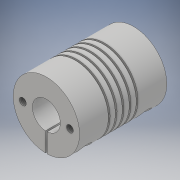
# Autodesk Inventor part: Муфта4х5
Saved by Autodesk Inventor 2017 (Build 210142000, 142)
## iProperties
Part Number: Муфта4х5
Material: Типовые
Document SubType Name: Modeling
Designer: Daemon
Density: 1 g/cm^3
Appearance: По умолчанию
Author: Daemon
Autodesk Inventor part; units mm, degrees
sketch "Эскиз1" plane through (0, 0, 0) normal (0, 0, 1) x (1, 0, 0)
  circle A0 centre (0, 0) radius 9.5
  dimension "d0" = 19
  constraints: 1 centre point, 1 coincident
  measures "d0" diameter of A0
extrude "Выдавливание1" add sketch "Эскиз1" along normal blind 25
sketch "Эскиз2" plane through (0, 0, 25) normal (0, 0, 1) x (1, 0, 0)
  circle A0 centre (0, 0) radius 3
  dimension "d3" = 6
  constraints: 1 centre point, 1 coincident
  measures "d3" diameter of A0
extrude "Выдавливание2" cut sketch "Эскиз2" against normal blind 12.5
sketch "Эскиз3" plane through (0, 0, 0) normal (0, 0, -1) x (-1, 0, 0)
  circle A0 centre (0, 0) radius 4
  dimension "d6" = 8
  constraints: 1 centre point, 1 coincident
  measures "d6" diameter of A0
extrude "Выдавливание3" cut sketch "Эскиз3" against normal blind 12.5
ref_plane "РабПлоскость1" through (-9.5, 0, 0) normal (1, 0, 0) x (0, 1, 0)
ref_plane "РабПлоскость2" through (0, 0, 12.5) normal (0, 0, -1) x (-1, 0, 0)
sketch "Эскиз5" plane through (0, 0, 12.5) normal (0, 0, -1) x (-1, 0, 0)
  circle A0 centre (0, 0) radius 9.5
  circle A1 centre (0, 0) radius 6.75
  dimension "d20" = 19
  dimension "d21" = 13.5
  constraints: 2 centre point, 2 coincident
  measures "d20" diameter of A0
  measures "d21" diameter of A1
extrude "Выдавливание5" cut sketch "Эскиз5" along normal mid plane 0.5
pattern_linear "Прямоуг.массив2" count 3 spacing 2 along (0, 0, 1) of "Выдавливание5"
pattern_linear "Прямоуг.массив3" count 3 spacing 2 along (0, 0, -1) of "Выдавливание5"
sketch "Эскиз6" plane through (0, 0, 0) normal (0, 0, -1) x (-1, 0, 0)
  circle A0 centre (0, 0) radius 9.5 projected
  circle A1 centre (0, 0) radius 6.75 projected
  line L0 (-9.5, 0.25) -> (-9.5, 0)
  line L1 (2, 0) -> (2, 0.25)
  line L2 (2, 0.25) -> (-9.5, 0.25)
  line L3 (2, 0) -> (-9.5, 0)
  dimension "d49" = 11.5
  dimension "d50" = 0.25
  constraints: 8 end point, 1 horizontal, 1 horizontal alignment, 1 perpendicular, 1 other
  measures "d49" distance of L1.start L0.end
  measures "d50" distance of L1.start L1.end
extrude "Выдавливание6" cut sketch "Эскиз6" against normal up to next contours L0 L2 A0 | A0 L2 A1 L3 | A1 L2 L1 L3 picked at (-7.6653, 0.1389) picked at (-0.9151, 0.1667)
sketch "Эскиз7" plane through (0, 0, 0) normal (0, 0, -1) x (-1, 0, 0)
  arc A0 (-6.75, 0) -> (-6.7454, 0.25) centre (0, 0) ccw projected
  circle A1 centre (0, 6.75) radius 1
  point P0 (6.7454, 0.25)
  dimension "d33" = 2
  constraints: 1 centre point, 1 point on circle
  measures "d33" diameter of A1
extrude "Выдавливание7" cut sketch "Эскиз7" against normal blind 4
pattern_circular "Круговой массив2" count 2 over 360 about axis through (0, 0, 0) along (0, 0, 1) of "Выдавливание7"
mirror "Зеркальное отражение2" about plane through (0, 0, 12.5) normal (0, 0, -1) of "Выдавливание7", "Круговой массив2"
thread "Резьба1" size "M2x0.4" class "6H" standard "ANSI Metric M Profile" full length
thread "Резьба2" size "M2x0.4" class "6H" standard "ANSI Metric M Profile" full length
thread "Резьба3" size "M2x0.4" class "6H" standard "ANSI Metric M Profile" full length
thread "Резьба4" size "M2x0.4" class "6H" standard "ANSI Metric M Profile" full length
mirror "Зеркальное отражение3" about plane through (-2, 0, 0) normal (0, 1, 0) of "Выдавливание6"
ref_plane "РабПлоскость3" through (0, -9.5, 0) normal (0, 1, 0) x (-1, 0, 0)
sketch "Эскиз8" plane through (0, -9.5, 0) normal (0, 1, 0) x (-1, 0, 0)
  line L0 (-9.5, -0.0521) -> (-9.5, 3.9479)
  line L1 (-9.5, 3.9479) -> (-7, 3.9479)
  circle A0 centre (-7, 3.9479) radius 1
  point P0 (0, 0)
  dimension "d51" = 2
  dimension "d52" = 2.5
  dimension "d53" = 4
  constraints: 4 end point, 1 centre point, 1 coincident, 1 horizontal, 1 vertical
  measures "d51" diameter of A0
  measures "d52" distance of L0.end L1.end
  measures "d53" distance of L0.start L0.end
extrude "Выдавливание8" cut sketch "Эскиз8" along normal up to next
sketch "Эскиз9" plane through (0, -9.5, 0) normal (0, 1, 0) x (-1, 0, 0)
  circle A0 centre (-7, 3.9479) radius 1 projected
  circle A1 centre (-7, 3.9479) radius 2
  point P0 (0, 0)
  dimension "d56" = 4
  constraints: 1 centre point, 1 coincident
  measures "d56" diameter of A1
extrude "Выдавливание9" cut sketch "Эскиз9" along normal blind 5
ref_plane "РабПлоскость5" through (0, 9.5, 0) normal (0, 1, 0) x (-1, 0, 0)
sketch "Эскиз10" plane through (0, 9.5, 0) normal (0, 1, 0) x (-1, 0, 0)
  circle A0 centre (-7, 3.9479) radius 1 projected
  circle A1 centre (-7, 3.9479) radius 1
  point P0 (0, 0)
  constraints: 1 centre point, 1 coincident
extrude "Выдавливание10" cut sketch "Эскиз10" against normal up to next
sketch "Эскиз11" plane through (0, 9.5, 0) normal (0, 1, 0) x (-1, 0, 0)
  circle A0 centre (-7, 3.9479) radius 1 projected
  circle A1 centre (-7, 3.9479) radius 2
  point P0 (0, 0)
  constraints: 1 centre point, 1 coincident
extrude "Выдавливание11" cut sketch "Эскиз11" against normal blind 5
mirror "Зеркальное отражение10" about plane through (0, 0, 12.5) normal (0, 0, -1) of "Выдавливание8", "Выдавливание9"
mirror "Зеркальное отражение11" about plane through (0, 0, 12.5) normal (0, 0, -1) of "Выдавливание10", "Выдавливание11"
